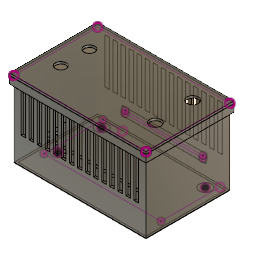
psuboardcase (Autodesk Fusion 360 design; units mm, degrees)
Autodesk Fusion 360 part; units mm, degrees
note: some values were not read from the file. Chosen so that the rebuilt part matches the saved one: which bodies a step acts on.
sketch "Sketch1" plane through (0, 0, 0) normal (0, 0, 1) x (1, 0, 0) in component "Board"
  line L0 (0, 0) -> (77.77, 0)
  line L1 (77.77, 0) -> (77.77, -39.2)
  line L2 (77.77, -39.2) -> (0, -39.2)
  line L3 (0, -39.2) -> (0, 0)
  line L4 (13.14, 0) -> (64.94, 0)
  line L5 (64.94, 0) -> (64.94, 11.2)
  line L6 (64.94, 11.2) -> (13.14, 11.2)
  line L7 (13.14, 11.2) -> (13.14, 0)
  circle A0 centre (4.125, -5.025) radius 1.625
  circle A1 centre (73.145, -5.125) radius 1.625
  circle A2 centre (4.125, -33.775) radius 1.625
  dimension "d1" = 77.77
  dimension "d2" = 39.2
  dimension "d3" = 51.8
  dimension "d4" = 11.2
  dimension "d5" = 13.14
  dimension "d6" = 12.83
  dimension "d7" = 3.25
  dimension "d8" = 3.25
  dimension "d9" = 3.25
  dimension "d10" = 4.125
  dimension "d11" = 5.425
  dimension "d12" = 4.125
  dimension "d13" = 5.025
  dimension "d14" = 4.625
  dimension "d15" = 5.125
  measures "d1" distance of L0.start L0.end
  measures "d2" distance of L0.start L2.end
  measures "d3" distance of L4.start L4.end
  measures "d4" distance of L4.start L6.end
  measures "d5" distance of L3 L7
  measures "d6" distance of L1 L5
  measures "d7" diameter of A0
  measures "d8" diameter of A1
  measures "d9" diameter of A2
  measures "d10" distance of L3 A2.centre
  measures "d11" distance of L2 A2.centre
  measures "d12" distance of L3 A0.centre
  measures "d13" distance of L0 A0.centre
  measures "d14" distance of L1 A1.centre
  measures "d15" distance of L0 A1.centre
extrude "Extrude1" add sketch "Sketch1" along normal blind 1.7 makes body 1 in component "Board"
ref_plane "WorkPlane1" through (38.885, -14, -9.3) normal (0, 0, 1) x (1, 0, 0) in component "Case"
sketch "Sketch1 (2)" plane through (38.885, -14, -9.3) normal (0, 0, 1) x (1, 0, 0) in component "Case"
  line L0 (-43.885, -40.2) -> (43.885, -40.2)
  line L1 (43.885, -40.2) -> (43.885, 15.5)
  line L2 (43.885, 15.5) -> (-43.885, 15.5)
  line L3 (-43.885, 15.5) -> (-43.885, -40.2)
  line L4 (-38.885, -25.2) -> (38.885, -25.2)
  line L5 (-38.885, 14) -> (-38.885, -25.2)
  line L6 (38.885, -25.2) -> (38.885, 14)
  line L7 (-25.745, 14) -> (-38.885, 14)
  line L8 (-42.485, 14.1) -> (-42.485, -38.8)
  line L9 (-42.485, -38.8) -> (42.485, -38.8)
  line L10 (42.485, -38.8) -> (42.485, 14.1)
  line L11 (42.485, 14.1) -> (-42.485, 14.1)
  circle A0 centre (-34.76, 8.975) radius 1.625
  circle A1 centre (-34.76, -19.775) radius 1.625
  circle A2 centre (34.26, 8.875) radius 1.625
  circle A3 centre (-34.76, 8.975) radius 4
  circle A4 centre (34.26, 8.875) radius 4
  circle A5 centre (-34.76, -19.775) radius 4
  circle A6 centre (-34.76, 8.975) radius 1
  circle A7 centre (34.26, 8.875) radius 1
  circle A8 centre (-34.76, -19.775) radius 1
  dimension "d19" = 15
  dimension "d20" = 5
  dimension "d21" = 5
  dimension "d22" = 1.5
  dimension "d23" = 1.4
  dimension "d24" = 8
  dimension "d25" = 8
  dimension "d26" = 8
  dimension "d29" = 2
  dimension "d30" = 2
  dimension "d31" = 2
  measures "d19" distance of L0 L4
  measures "d20" distance of L3 L5
  measures "d21" distance of L1 L6
  measures "d22" distance of L2 L7
  measures "d24" diameter of A3
  measures "d25" diameter of A4
  measures "d26" diameter of A5
  measures "d29" diameter of A6
  measures "d30" diameter of A7
  measures "d31" diameter of A8
extrude "Extrude1'" add sketch "Sketch1 (2)" along normal up to surface (9.3 mm away) separate body contours A0 | A1 | A2 | A3 | A4 | A5 makes body 2 at (8.12, -5.2244, -3.1) makes body 3 at (77.14, -5.3244, -3.1) makes body 4 at (8.12, -33.9744, -3.1) in component "Case"
extrude "Extrude2" add sketch "Sketch1 (2)" along normal blind 50 separate body contours L0 L1 L2 L3 makes body 5 in component "Case"
sketch "Sketch2" plane through (0, 1.5, 0) normal (0, 1, 0) x (-1, 0, 0) in component "Case"
  line L0 (-82.77, -9.3) -> (5, -9.3)
  line L1 (5, -9.3) -> (5, 40.7)
  line L2 (5, 40.7) -> (-82.77, 40.7)
  line L3 (-82.77, 40.7) -> (-82.77, -9.3)
  line L4 (-64.94, 0) -> (-13.14, 0)
  line L5 (-13.14, 0) -> (-13.14, 1.7)
  line L6 (-13.14, 1.7) -> (-64.94, 1.7)
  line L7 (-64.94, 1.7) -> (-64.94, 0)
  line L8 (-66.94, -2) -> (-11.14, -2)
  line L9 (-11.14, -2) -> (-11.14, 3.7)
  line L10 (-11.14, 3.7) -> (-66.94, 3.7)
  line L11 (-66.94, 3.7) -> (-66.94, -2)
  line L12 (-77.77, 38.7) -> (-74.77, 38.7)
  line L13 (-74.77, 38.7) -> (-74.77, 8.7)
  line L14 (-74.77, 8.7) -> (-77.77, 8.7)
  line L15 (-77.77, 8.7) -> (-77.77, 38.7)
  line L16 (-69.4129, 38.7) -> (-69.4129, 8.7)
  line L17 (-72.4129, 8.7) -> (-72.4129, 38.7)
  line L18 (-72.4129, 38.7) -> (-69.4129, 38.7)
  line L19 (-69.4129, 8.7) -> (-72.4129, 8.7)
  line L20 (-64.0557, 38.7) -> (-64.0557, 8.7)
  line L21 (-67.0557, 8.7) -> (-67.0557, 38.7)
  line L22 (-67.0557, 38.7) -> (-64.0557, 38.7)
  line L23 (-64.0557, 8.7) -> (-67.0557, 8.7)
  line L24 (-58.6986, 38.7) -> (-58.6986, 8.7)
  line L25 (-61.6986, 8.7) -> (-61.6986, 38.7)
  line L26 (-61.6986, 38.7) -> (-58.6986, 38.7)
  line L27 (-58.6986, 8.7) -> (-61.6986, 8.7)
  line L28 (-53.3414, 38.7) -> (-53.3414, 8.7)
  line L29 (-56.3414, 8.7) -> (-56.3414, 38.7)
  line L30 (-56.3414, 38.7) -> (-53.3414, 38.7)
  line L31 (-53.3414, 8.7) -> (-56.3414, 8.7)
  line L32 (-47.9843, 38.7) -> (-47.9843, 8.7)
  line L33 (-50.9843, 8.7) -> (-50.9843, 38.7)
  line L34 (-50.9843, 38.7) -> (-47.9843, 38.7)
  line L35 (-47.9843, 8.7) -> (-50.9843, 8.7)
  line L36 (-42.6271, 38.7) -> (-42.6271, 8.7)
  line L37 (-45.6271, 8.7) -> (-45.6271, 38.7)
  line L38 (-45.6271, 38.7) -> (-42.6271, 38.7)
  line L39 (-42.6271, 8.7) -> (-45.6271, 8.7)
  line L40 (-37.27, 38.7) -> (-37.27, 8.7)
  line L41 (-40.27, 8.7) -> (-40.27, 38.7)
  line L42 (-40.27, 38.7) -> (-37.27, 38.7)
  line L43 (-37.27, 8.7) -> (-40.27, 8.7)
  line L44 (-31.9129, 38.7) -> (-31.9129, 8.7)
  line L45 (-34.9129, 8.7) -> (-34.9129, 38.7)
  line L46 (-34.9129, 38.7) -> (-31.9129, 38.7)
  line L47 (-31.9129, 8.7) -> (-34.9129, 8.7)
  line L48 (-26.5557, 38.7) -> (-26.5557, 8.7)
  line L49 (-29.5557, 8.7) -> (-29.5557, 38.7)
  line L50 (-29.5557, 38.7) -> (-26.5557, 38.7)
  line L51 (-26.5557, 8.7) -> (-29.5557, 8.7)
  line L52 (-21.1986, 38.7) -> (-21.1986, 8.7)
  line L53 (-24.1986, 8.7) -> (-24.1986, 38.7)
  line L54 (-24.1986, 38.7) -> (-21.1986, 38.7)
  line L55 (-21.1986, 8.7) -> (-24.1986, 8.7)
  line L56 (-15.8414, 38.7) -> (-15.8414, 8.7)
  line L57 (-18.8414, 8.7) -> (-18.8414, 38.7)
  line L58 (-18.8414, 38.7) -> (-15.8414, 38.7)
  line L59 (-15.8414, 8.7) -> (-18.8414, 8.7)
  line L60 (-10.4843, 38.7) -> (-10.4843, 8.7)
  line L61 (-13.4843, 8.7) -> (-13.4843, 38.7)
  line L62 (-13.4843, 38.7) -> (-10.4843, 38.7)
  line L63 (-10.4843, 8.7) -> (-13.4843, 8.7)
  line L64 (-5.1271, 38.7) -> (-5.1271, 8.7)
  line L65 (-8.1271, 8.7) -> (-8.1271, 38.7)
  line L66 (-8.1271, 38.7) -> (-5.1271, 38.7)
  line L67 (-5.1271, 8.7) -> (-8.1271, 8.7)
  line L68 (0.23, 38.7) -> (0.23, 8.7)
  line L69 (-2.77, 8.7) -> (-2.77, 38.7)
  line L70 (-2.77, 38.7) -> (0.23, 38.7)
  line L71 (0.23, 8.7) -> (-2.77, 8.7)
  dimension "d34" = 2
  dimension "d39" = 30
  dimension "d40" = 3
  dimension "d41" = 5
  dimension "d42" = 2
  dimension "d45" = 75
  dimension "d46" = 0
  measures "d39" distance of L12.start L14.end
  measures "d40" distance of L12.start L12.end
  measures "d41" distance of L3 L15
  measures "d42" distance of L2 L12
extrude "Extrude3" cut sketch "Sketch2" against normal blind 5 contours L4 L5 L6 L7 | L8 L9 L10 L11 bodies 5 in component "Case"
extrude "Extrude4" add sketch "Sketch1 (2)" along normal blind 1.5 contours L8 L9 L10 L11 bodies 4 2 3 5 in component "Case"
extrude "Extrude5" cut sketch "Sketch2" against normal blind 79 contours L12 L13 L14 L15 | L16 L17 L18 L19 | L20 L21 L22 L23 | L24 L25 L26 L27 | L28 L29 L30 L31 | L32 L33 L34 L35 | L36 L37 L38 L39 | L40 L41 L42 L43 | L44 L45 L46 L47 | L48 L49 L50 L51 | L52 L53 L54 L55 | L56 L57 L58 L59 | L60 L61 L62 L63 | L64 L65 L66 L67 | L68 L69 L70 L71 bodies 4 in component "Case"
sketch "Sketch1 (3)" plane through (0, 0, 40.7) normal (0, 0, 1) x (-1, 0, 0) in component "Component"
  line L0 (3.6, -0.1) -> (-81.37, -0.1)
  line L1 (-81.37, -0.1) -> (-81.37, 52.8)
  line L2 (-81.37, 52.8) -> (3.6, 52.8)
  line L3 (3.6, 52.8) -> (3.6, -0.1)
  line L4 (5, -1.5) -> (5, 54.2)
  line L5 (5, 54.2) -> (-82.77, 54.2)
  line L6 (-82.77, 54.2) -> (-82.77, -1.5)
  line L7 (-82.77, -1.5) -> (5, -1.5)
  line L8 (5, -1.5) -> (5, 54.2)
  line L9 (-82.77, -1.5) -> (5, -1.5)
  line L10 (-82.77, 54.2) -> (-82.77, -1.5)
  line L11 (5, 54.2) -> (-82.77, 54.2)
  line L12 (-84.27, 55.7) -> (-84.27, -3)
  line L13 (-84.27, -3) -> (6.5, -3)
  line L14 (6.5, -3) -> (6.5, 55.7)
  line L15 (6.5, 55.7) -> (-84.27, 55.7)
  dimension "d49" = 1.5
extrude "Extrude1''" add sketch "Sketch1 (3)" against normal blind 5 separate body contours L12 L13 L14 L15 makes body 6 in component "Component"
extrude "Extrude2'" add sketch "Sketch1 (3)" along normal blind 1.5 contours L0 L1 L2 L3 | L4 L5 L6 L7 L8 L9 L10 L11 | L12 L13 L14 L15 bodies 6 in component "Component"
sketch "Sketch2 (2)" plane through (0, 0, 42.2) normal (0, 0, 1) x (-1, 0, 0) in component "Component"
  line L0 (6.5, 55.7) -> (-84.27, 55.7)
  line L1 (-84.27, 55.7) -> (-84.27, -3)
  line L2 (-84.27, -3) -> (6.5, -3)
  line L3 (6.5, -3) -> (6.5, 55.7)
  circle A0 centre (-6.4353, 15.4556) radius 3.5
  circle A1 centre (-6.4353, 34.5056) radius 3.5
  line L4 (-6.4353, 34.5056) -> (-6.4353, 15.4556)
  circle A2 centre (-70.1327, 10.5128) radius 3.8
  circle A3 centre (-70.6962, 35.8899) radius 3.8
  dimension "d54" = 7
  dimension "d55" = 7
  dimension "d56" = 19.05
  dimension "d57" = 7.6
  dimension "d58" = 7.6
  measures "d54" diameter of A0
  measures "d55" diameter of A1
  measures "d56" distance of A0.centre A1.centre
  measures "d57" diameter of A2
  measures "d58" diameter of A3
extrude "Extrude3'" cut sketch "Sketch2 (2)" against normal blind 2 contours A0 | A1 | A2 | A3 bodies 6 in component "Component"
component "Board" placed x (1, 0, 0) y (0, 1, 0) z (0, 0, 1) at (0, 0, 0)
component "Case" placed x (1, 0, 0) y (0, 1, 0) z (0, 0, 1) at (0, 0, 0)
component "Component" placed x (1, 0, 0) y (0, 1, 0) z (0, 0, 1) at (0, 0, 0)
equation "d10 = 2.5 mm + ( 3.25 / 2 ) * 1 mm"
equation "d11 = 3.8 mm + ( 3.25 / 2 ) * 1 mm"
equation "d13 = 3.4 mm + ( 3.25 / 2 ) * 1 mm"
equation "d14 = 3 mm + ( 3.25 / 2 ) * 1 mm"
equation "d15 = 3.5 mm + ( 3.25 / 2 ) * 1 mm"
